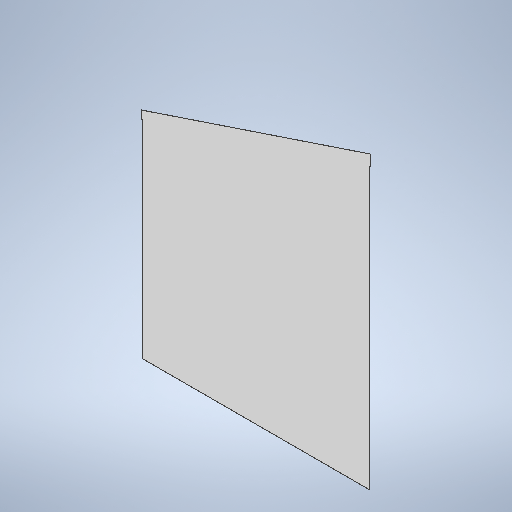
# Autodesk Inventor part: Underlayment_For_Side
Saved by Autodesk Inventor 2025 (Build 290162010, 162A)
## iProperties
Created: 2024-10-02
Part Number: Underlayment_For_Side
Material: Generic
Document SubType Name: Modeling
Designer: Tom
Density: 1 g/cm^3
Appearance: White
Author: Tom
Autodesk Inventor part; units mm, degrees
ref_plane "YZ Plane" through (0, 0, 0) normal (1, 0, 0) x (0, 1, 0)
ref_plane "XZ Plane" through (0, 0, 0) normal (0, 1, 0) x (-1, 0, 0)
ref_plane "XY Plane" through (0, 0, 0) normal (0, 0, 1) x (1, 0, 0)
sketch "Sketch1" plane through (0, 0, 0) normal (0, 0, 1) x (1, 0, 0)
  line L0 (0, 0) -> (0, 3086.1)
  line L1 (0, 3086.1) -> (-17.6276, 3086.1)
  line L2 (-17.6276, 3086.1) -> (-17.6276, 3205.0228)
  line L3 (0, 0) -> (3394.075, 0)
  line L4 (3394.075, 0) -> (3394.075, 4185.2342)
  line L5 (3394.075, 4185.2342) -> (3413.3028, 4185.2342)
  line L6 (3413.3028, 4185.2342) -> (3413.3028, 4349.242)
  line L7 (3413.3028, 4349.242) -> (-17.6276, 3205.0228)
  dimension "d1" = 3086.1
  dimension "d2" = 17.6276
  dimension "d3" = 118.9228
  dimension "d4" = 3394.075
  dimension "d5" = 4185.2342
  dimension "d6" = 19.2278
  dimension "d7" = 164.0078
  constraints: 16 end point, 4 vertical, 3 horizontal
  measures "d1" distance of L0.start L0.end
  measures "d2" distance from line of L0 L1.end
  measures "d3" distance of L1.end L2.end
  measures "d4" distance of L0.start L3.end
  measures "d5" distance of L3.end L4.end
  measures "d6" distance of L4.end L5.end
  measures "d7" distance of L5.end L6.end
extrude "Extrusion1" add sketch "Sketch1" along normal blind 1.5875
body "Solid1"
